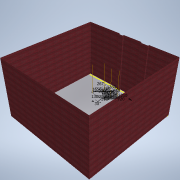
# Autodesk Inventor part: Entorno
Saved by Autodesk Inventor 2020 (Build 240168000, 168)
## iProperties
Created: 2019-10-05
Part Number: Entorno
Material: Genérico
Document SubType Name: Modeling
Designer: dasa1
Density: 1 g/cm^3
Appearance: Textura gruesa - Blanco
Author: dasa1
Autodesk Inventor part; units mm, degrees
ref_plane "YZ Plane" through (0, 0, 0) normal (1, 0, 0) x (0, 1, 0)
ref_plane "XZ Plane" through (0, 0, 0) normal (0, 1, 0) x (-1, 0, 0)
ref_plane "XY Plane" through (0, 0, 0) normal (0, 0, 1) x (1, 0, 0)
sketch "Boceto1" plane through (0, 0, 0) normal (0, 1, 0) x (-1, 0, 0)
  line L0 (0, 0) -> (0, -650) construction
  line L1 (0, -650) -> (4000, -650) construction
  line L2 (4000, -650) -> (-6000, -650)
  line L3 (-6000, -650) -> (-6000, 9350)
  line L4 (-6000, 9350) -> (4000, 9350)
  line L5 (4000, 9350) -> (4000, -650)
  dimension "d1" = 650
  dimension "d2" = 4000
  dimension "d3" = 10000
  dimension "d4" = 10000
  constraints: 12 end point, 2 parallel, 2 perpendicular, 1 horizontal, 1 vertical
  measures "d1" distance of L0.start L0.end
  measures "d2" distance of L0.end L1.end
  measures "d3" distance of L3.end L4.end
  measures "d4" distance of L2.end L3.end
extrude "Extrusión1" add sketch "Boceto1" along normal blind 1
sketch "Boceto3" plane through (0, 1, 0) normal (0, 1, 0) x (1, 0, 0)
  line L0 (-4000, 650) -> (-4000, -9350) construction
  line L1 (-4000, -9350) -> (6000, -9350) construction
  line L2 (6000, -9350) -> (6000, 650) construction
  line L3 (6000, 650) -> (-4000, 650) construction
  line L4 (6000, 650) -> (6000, 651)
  line L5 (-4000, 650) -> (-4000, -9350) projected
  line L6 (-4001, 650) -> (-4001, -9350)
  line L7 (-4001, -9350) -> (-4000, -9350)
  line L8 (-4000, -9350) -> (-4000, 650)
  line L9 (-4000, -9350) -> (6000, -9350)
  line L10 (6000, -9350) -> (6000, -9351)
  line L11 (6000, -9351) -> (-4000, -9351)
  line L12 (-4000, -9351) -> (-4000, -9350)
  line L13 (6000, -9350) -> (6001, -9350)
  line L14 (6001, -9350) -> (6001, 650)
  line L15 (6001, 650) -> (6000, 650) construction
  line L16 (6000, 650) -> (6000, -9350)
  line L17 (-50, 651) -> (200, 651)
  line L18 (200, 651) -> (-200, 651)
  line L19 (0, 651) -> (250, 651) construction
  line L20 (250, 651) -> (-249, 651) construction
  line L21 (-250, 651) -> (-249, 651) construction
  line L22 (-249, 651) -> (-249, 801)
  line L23 (-249, 801) -> (-250, 801)
  line L24 (-250, 800) -> (-250, 651)
  line L25 (250, 651) -> (249, 651) construction
  line L26 (249, 651) -> (249, 801)
  line L27 (249, 801) -> (250, 801)
  line L28 (250, 800) -> (250, 651)
  line L29 (249, 651) -> (-249, 651)
  line L30 (6000, 801) -> (6000, 800) construction
  line L31 (249, 800) -> (249, 801)
  line L32 (6001, 650) -> (6000, 650) construction
  line L33 (6000, 650) -> (6000, 800)
  line L34 (6000, 800) -> (6001, 800) construction
  line L35 (6001, 800) -> (6001, 650)
  line L36 (-250, 801) -> (-4000, 801)
  line L37 (-4000, 801) -> (-4000, 800) construction
  line L38 (-4000, 800) -> (-250, 800)
  line L39 (-250, 800) -> (-250, 801) construction
  line L40 (-4000, 801) -> (-4001, 801)
  line L41 (-4001, 801) -> (-4001, 650)
  line L42 (-4000, 651) -> (-4000, 800)
  line L43 (-250, 651) -> (-250, 650)
  line L44 (250, 651) -> (250, 650)
  line L45 (6000, 650) -> (-4000, 650) projected
  line L46 (6000, 801) -> (6001, 801)
  line L47 (6001, 801) -> (6001, 800)
  line L48 (6001, 800) -> (6000, 800) construction
  line L49 (6000, 800) -> (6000, 801) construction
  line L50 (2210, 650) -> (2210, 200) construction
  line L51 (2210, 200) -> (3040, 200) construction
  line L52 (3040, 200) -> (3040, 650) construction
  line L53 (3040, 650) -> (2210, 650) construction
  line L54 (2210, 650) -> (2211, 650)
  line L55 (2211, 651) -> (2211, 800)
  line L56 (2211, 800) -> (2210, 800) construction
  line L57 (2210, 800) -> (2210, 650)
  line L58 (3040, 650) -> (3039, 650)
  line L59 (3039, 651) -> (3039, 800)
  line L60 (3039, 800) -> (3040, 800) construction
  line L61 (3040, 800) -> (3040, 650)
  line L62 (2211, 650) -> (3039, 650)
  line L63 (3039, 650) -> (3039, 651) construction
  line L64 (3039, 651) -> (2211, 651)
  line L65 (2211, 651) -> (2211, 650) construction
  line L66 (2210, 800) -> (250, 800)
  line L67 (6000, 800) -> (3040, 800)
  line L68 (2211, 801) -> (2211, 800)
  line L69 (3039, 800) -> (3039, 801)
  line L70 (249, 801) -> (2211, 801)
  line L71 (3039, 801) -> (6000, 801)
  line L72 (-4000, 651) -> (-4000, 650)
  point P0 (0, 0)
  point P1 (-4000, -9350)
  point P2 (-4000, -9350)
  point P3 (-2000, -9350)
  point P4 (6000, 650)
  point P5 (6000, 650)
  dimension "d7" = 1
  dimension "d8" = 1
  dimension "d9" = 1
  dimension "d10" = 1
  dimension "d24" = 10000
  dimension "d32" = 0
  dimension "d34" = 0
  dimension "d36" = 10000
  dimension "d37" = 8000
  dimension "d38" = 10000
  dimension "d39" = 8000
  dimension "d40" = 10000
  dimension "d41" = 8000
  dimension "d42" = 0
  dimension "d81" = 250
  dimension "d82" = 500
  dimension "d83" = 1
  dimension "d84" = 150
  dimension "d85" = 1
  dimension "d86" = 150
  dimension "d87" = 1
  dimension "d88" = 1
  dimension "d89" = 90
  dimension "d90" = 90
  dimension "d94" = 0
  dimension "d95" = 0
  dimension "d96" = 151
  dimension "d97" = 5751
  dimension "d98" = 4250
  dimension "d99" = 0
  dimension "d100" = 1
  dimension "d101" = 0
  dimension "d102" = 0
  dimension "d103" = 150
  dimension "d104" = 5800
  dimension "d105" = 6050
  dimension "d106" = 0
  dimension "d107" = 1
  dimension "d108" = 0
  dimension "d111" = 1
  dimension "d112" = 1
  dimension "d113" = 1
  dimension "d114" = 90
  dimension "d115" = 151
  dimension "d116" = 150
  dimension "d117" = 2961
  constraints: 134 end point, 28 parallel, 16 perpendicular, 13 horizontal, 4 point on line, 1 collinear, 1 midpoint, 2 other
  measures "d7" distance of L4.end L4.start
  measures "d8" distance of L7.end L6.end
  measures "d9" distance of L9.end L10.end
  measures "d10" distance of L15.end L14.end
  measures "d24" distance between parallel lines of L3 L7
  measures "d32" distance from line of point (6000, 650) L3
  measures "d34" distance from line of point (6000, 650) L3
  measures "d36" distance from line of point (-4000, -9350) L3
  measures "d38" distance from line of point (-4000, -9350) L3
  measures "d40" distance from line of point (-2000, -9350) L3
  measures "d41" distance from line of point (-2000, -9350) L2
  measures "d42" distance between parallel lines of L2 L16
  measures "d81" distance of L19.start L19.end
  measures "d82" distance of L19.end L21.start
  measures "d83" distance of L23.end L22.end
  measures "d84" distance of L20.end L22.end
  measures "d85" distance of L26.end L27.end
  measures "d86" distance of L25.end L26.end
  measures "d87" distance of L30.start L30.end
  measures "d88" distance of L37.end L36.end
  measures "d89" angle to the sketch x axis of L44
  measures "d90" angle to the sketch x axis of L8
  measures "d94" vertical extent of L32
  measures "d95" distance between parallel lines of L2 L30
  measures "d96" distance between parallel lines of L3 L27
  measures "d97" distance between parallel lines of L2 L26
  measures "d98" distance between parallel lines of L0 L28
  measures "d99" distance between parallel lines of L0 L42
  measures "d100" distance from line of L4.end L3
  measures "d101" distance from line of point (6000, 650) L2
  measures "d102" distance from line of point (6000, 650) L2
  measures "d103" distance from line of L31.start L3
  measures "d104" distance from line of L17.end L2
  measures "d105" distance from line of L17.start L2
  measures "d106" distance from line of L43.end L3
  measures "d107" distance from line of L42.start L3
  measures "d108" distance from line of L6.start L3
  measures "d111" distance of L56.end L55.end
  measures "d112" distance of L59.end L60.end
  measures "d113" distance of L59.start L62.end
  measures "d114" angle of L53 L4
  measures "d115" distance between parallel lines of L53 L46
  measures "d116" distance between parallel lines of L53 L66
  measures "d117" distance from line of L58.end L2
extrude "Extrusión2" add sketch "Boceto3" along normal blind 6000 contours L4 L33 L67 L61 L45 L57 L66 L28 L44 L43 L24 L38 L42 L72 L5 L7 L6 L41 L40 L36 L23 L22 L29 L18 L17 L26 L27 L70 L68 L55 L64 L59 L69 L71 L46 L47 L35 L14 L13 L16 | L10 L11 L12 L9
sketch "Boceto4" plane through (0, 1, 0) normal (0, 1, 0) x (1, 0, 0)
  line L0 (0, 0) -> (370, 0) construction
  line L1 (0, 0) -> (2210, 0) construction
  line L2 (0, 0) -> (-385, 0) construction
  line L3 (0, 185) -> (0, 0) construction
  line L4 (0, 0) -> (-1260, 0) construction
  line L5 (0, 360) -> (0, 0) construction
  line L6 (0, 0) -> (250, 0) construction
  line L7 (250, 0) -> (250, -820) construction
  line L8 (250, -820) -> (0, -820) construction
  line L9 (0, -820) -> (0, 0) construction
  line L10 (0, 0) -> (-300, 0) construction
  line L11 (-300, 0) -> (-300, -1247) construction
  line L12 (-300, -1247) -> (0, -1247) construction
  line L13 (0, -1247) -> (0, 0) construction
  line L14 (0, 0) -> (30, 0) construction
  line L15 (30, 0) -> (30, -2220) construction
  line L16 (30, -2220) -> (0, -2220) construction
  line L17 (0, -2220) -> (0, 0) construction
  line L18 (0, 0) -> (1200, 0) construction
  line L19 (1200, 0) -> (1200, -720) construction
  line L20 (1200, -720) -> (0, -720) construction
  line L21 (0, -720) -> (0, 0) construction
  line L22 (0, 0) -> (-650, 0) construction
  line L23 (-650, 0) -> (-650, -650) construction
  line L24 (-650, -650) -> (0, -650) construction
  line L25 (0, -650) -> (0, 0) construction
  line L26 (6000, 650) -> (-4000, 650) projected
  line L27 (0, 0) -> (-1300, 0) construction
  line L28 (-1300, 0) -> (-1300, -1650) construction
  line L29 (-1300, -1650) -> (0, -1650) construction
  line L30 (0, -1650) -> (0, 0) construction
  line L31 (0, 0) -> (515, 0) construction
  line L32 (515, 0) -> (515, -1475) construction
  line L33 (515, -1475) -> (0, -1475) construction
  line L34 (0, -1475) -> (0, 0) construction
  line L35 (0, 0) -> (485, 0) construction
  line L36 (485, 0) -> (485, -1240) construction
  line L37 (485, -1240) -> (0, -1240) construction
  line L38 (0, -1240) -> (0, 0) construction
  line L39 (0, 0) -> (495, 0) construction
  line L40 (495, 0) -> (495, -972) construction
  line L41 (495, -972) -> (0, -972) construction
  line L42 (0, -972) -> (0, 0) construction
  line L43 (0, 0) -> (-385, 0) construction
  line L44 (-385, 0) -> (-385, -185) construction
  line L45 (-385, -185) -> (0, -185) construction
  line L46 (0, -185) -> (0, 0) construction
  line L47 (0, 0) -> (-1360, 0) construction
  line L48 (-1360, 0) -> (-1360, 267) construction
  line L49 (-1360, 267) -> (0, 267) construction
  line L50 (0, 267) -> (0, 0) construction
  line L51 (30, 0) -> (3030, 0) construction
  line L52 (0, 0) -> (-1414.2136, -1414.2136)
  line L53 (0, 0) -> (2000, 0) construction
  line L54 (0, 0) -> (30, -33.541)
  line L55 (30, -33.541) -> (-33.6396, 30.0986)
  line L56 (-33.6396, 30.0986) -> (-1447.8532, -1384.115)
  line L57 (-385, -185) -> (-1360, 0) construction
  point P0 (0, 650)
  dimension "d13" = 370
  dimension "d14" = 2210
  dimension "d19" = 250
  dimension "d20" = 820
  dimension "d21" = 300
  dimension "d22" = 1247
  dimension "d47" = 30
  dimension "d48" = 2220
  dimension "d49" = 1200
  dimension "d50" = 720
  dimension "d51" = 650
  dimension "d52" = 650
  dimension "d54" = 650
  dimension "d56" = 1300
  dimension "d57" = 1650
  dimension "d58" = 515
  dimension "d59" = 1475
  dimension "d60" = 485
  dimension "d61" = 1240
  dimension "d62" = 495
  dimension "d63" = 972
  dimension "d64" = 385
  dimension "d65" = 185
  dimension "d66" = 1360
  dimension "d67" = 267
  dimension "d70" = 2000
  dimension "d71" = 135
  dimension "d72" = 45
  dimension "d73" = 90
  dimension "d74" = 2000
  constraints: 82 end point, 30 horizontal, 22 parallel, 13 perpendicular, 13 vertical, 2 point on line, 1 coincident, 1 horizontal alignment, 6 other
  measures "d19" distance of L7.end L8.end
  measures "d20" distance of L6.end L7.end
  measures "d21" distance of L12.end L11.end
  measures "d22" distance of L11.end L10.end
  measures "d47" distance of L15.end L16.end
  measures "d48" distance of L14.end L15.end
  measures "d49" distance of L19.end L20.end
  measures "d50" distance of L18.end L19.end
  measures "d51" distance of L24.end L23.end
  measures "d52" distance of L23.end L22.end
  measures "d56" distance of L29.end L28.end
  measures "d57" distance of L28.end L27.end
  measures "d58" distance of L32.end L33.end
  measures "d59" distance of L31.end L32.end
  measures "d60" distance of L36.end L37.end
  measures "d61" distance of L35.end L36.end
  measures "d62" distance of L40.end L41.end
  measures "d63" distance of L39.end L40.end
  measures "d64" distance of L45.end L44.end
  measures "d65" distance of L44.end L43.end
  measures "d66" distance of L48.end L49.end
  measures "d67" distance of L47.end L48.end
  measures "d71" angle of L52 L53
  measures "d73" distance of L54.end L55.end
  measures "d74" distance of L55.end L56.end
sketch "Boceto5" plane through (0, 0, 0) normal (0, -1, 0) x (1, 0, 0)
  line L0 (-249, -801) -> (-4001, -801) projected
  line L1 (-249, -651) -> (-249, -801) projected
  line L2 (250, -650) -> (250, -800) projected
  line L3 (250, -800) -> (2210, -800) projected
  line L4 (2210, -800) -> (2210, -650) projected
  line L5 (6001, -801) -> (3039, -801) projected
  line L6 (3039, -801) -> (3039, -651) projected
  line L7 (6000, -800) -> (6000, -650) projected
  line L8 (-4000, -650) -> (-4000, -800) projected
  line L9 (6000, -650) -> (-4000, -650) projected
  line L10 (6001, -801) -> (3039, -801) projected
  line L11 (6000, -650) -> (3040, -650) projected
  line L12 (6001, -801) -> (3040, -801)
  line L13 (3040, -801) -> (3040, -650)
  line L14 (3040, -650) -> (6001, -650)
  line L15 (6001, -650) -> (6001, -801)
  line L16 (250, -800) -> (2210, -800) projected
  line L17 (249, -801) -> (249, -651) projected
  line L18 (2210, -800) -> (249, -800)
  line L19 (249, -800) -> (249, -651)
  line L20 (249, -651) -> (2210, -651)
  line L21 (2210, -651) -> (2210, -800)
  line L22 (-250, -650) -> (-4000, -650) projected
  line L23 (-249, -801) -> (-4000, -801)
  line L24 (-4000, -801) -> (-4000, -650)
  line L25 (-4000, -650) -> (-249, -650)
  line L26 (-249, -650) -> (-249, -801)
  point P0 (0, 0)
  point P1 (-249, -650)
  constraints: 24 end point, 6 parallel, 3 horizontal, 3 perpendicular
extrude "Extrusión3" add sketch "Boceto5" against normal blind 1 contours L9 L14 L15 L5 L13 | L0 L24 L8 L9 L26 L1 | L20 L4 L3 L2 | L2 L18 L17 L20
sketch "Boceto6" plane through (-249, 1, -650) normal (0, 0, 1) x (1, 0, 0)
  line L0 (499, 0) -> (0, 0) construction
  line L1 (499, 0) -> (499, 6000) construction
  line L2 (-1, 6000) -> (499, 6000) construction
  line L3 (-1, 0) -> (-1, 6000) construction
  line L4 (0, 0) -> (-1, 0) construction
  line L5 (249, -1) -> (249, 2299) construction
  line L6 (249, 2299) -> (249, 2449) construction
  line L7 (249, 2449) -> (249, 2661.5) construction
  line L8 (249, 2449) -> (289, 2449) construction
  line L9 (289, 2449) -> (289, 2474) construction
  line L10 (289, 2474) -> (249, 2474) construction
  line L11 (249, 2474) -> (249, 2449) construction
  line L12 (289, 2474) -> (209, 2474)
  line L13 (209, 2474) -> (209, 2449)
  line L14 (209, 2449) -> (289, 2449)
  line L15 (289, 2449) -> (289, 2474)
  line L16 (249, 2274) -> (289, 2274) construction
  line L17 (289, 2274) -> (289, 2299) construction
  line L18 (289, 2299) -> (249, 2299) construction
  line L19 (249, 2299) -> (249, 2274) construction
  line L20 (289, 2299) -> (209, 2299)
  line L21 (209, 2299) -> (209, 2274)
  line L22 (209, 2274) -> (289, 2274)
  line L23 (289, 2274) -> (289, 2299)
  line L24 (249, 2661.5) -> (274, 2661.5) construction
  line L25 (274, 2661.5) -> (274, 2674) construction
  line L26 (274, 2674) -> (249, 2674) construction
  line L27 (249, 2674) -> (249, 2661.5) construction
  line L28 (274, 2674) -> (224, 2674)
  line L29 (224, 2674) -> (224, 2649)
  line L30 (224, 2649) -> (274, 2649)
  line L31 (274, 2649) -> (274, 2674)
  line L32 (249, 2086.5) -> (274, 2086.5) construction
  line L33 (274, 2086.5) -> (274, 2099) construction
  line L34 (274, 2099) -> (249, 2099) construction
  line L35 (249, 2099) -> (249, 2086.5) construction
  line L36 (274, 2099) -> (224, 2099)
  line L37 (224, 2099) -> (224, 2074)
  line L38 (224, 2074) -> (274, 2074)
  line L39 (274, 2074) -> (274, 2099)
  dimension "d120" = 2300
  dimension "d121" = 150
  dimension "d122" = 212.5
  dimension "d125" = 40
  dimension "d126" = 25
  dimension "d127" = 80
  dimension "d128" = 25
  dimension "d129" = 40
  dimension "d130" = 25
  dimension "d131" = 80
  dimension "d132" = 25
  dimension "d135" = 25
  dimension "d136" = 12.5
  dimension "d137" = 50
  dimension "d138" = 25
  dimension "d142" = 25
  dimension "d143" = 12.5
  dimension "d144" = 50
  dimension "d145" = 25
  dimension "d164" = 2274
  dimension "d165" = 2099
  dimension "d166" = 210
  dimension "d167" = 225
  constraints: 70 end point, 16 parallel, 8 horizontal, 8 perpendicular, 3 vertical, 1 coincident
  measures "d120" distance of L5.start L5.end
  measures "d121" distance of L5.end L6.end
  measures "d122" distance of L6.end L7.end
  measures "d125" distance of L10.end L9.end
  measures "d126" distance of L9.end L8.end
  measures "d127" distance of L14.end L13.end
  measures "d128" distance of L13.end L12.end
  measures "d129" distance of L18.end L17.end
  measures "d130" distance of L17.end L16.end
  measures "d131" distance of L22.end L22.start
  measures "d132" distance of L22.start L20.end
  measures "d135" distance of L26.end L25.end
  measures "d136" distance of L25.end L24.end
  measures "d137" distance of L30.end L29.end
  measures "d138" distance of L29.end L28.end
  measures "d142" distance of L35.start L36.start
  measures "d143" distance of L36.start L32.end
  measures "d144" distance of L38.end L38.start
  measures "d145" distance of L38.start L37.start
  measures "d164" distance between parallel lines of L0 L16
  measures "d165" distance between parallel lines of L0 L34
  measures "d166" distance between parallel lines of L1 L17
  measures "d167" distance between parallel lines of L1 L33
extrude "Extrusión4" add sketch "Boceto6" along normal blind 80 contours L15 L14 L13 L12 | L23 L22 L21 L20
ref_plane "Plano de trabajo1" through (0, 2450, -650) normal (1, 0, 0) x (0, 1, 0)
sketch "Boceto7" plane through (0, 2450, -650) normal (1, 0, 0) x (0, 1, 0)
  line L0 (-2449, 0) -> (3551, 0) construction
  line L1 (25, 0) -> (25, 80) construction
  line L2 (0, 0) -> (0, 80) construction
  line L3 (-150, 0) -> (-150, 80) construction
  line L4 (-175, 0) -> (-175, 80) construction
  line L5 (-150, 0) -> (-150, 650) construction
  line L6 (-150, 0) -> (500, 0) construction
  line L7 (-150, 650) -> (-150, 0) construction
  line L8 (225, 0) -> (200, 0) construction
  line L9 (25, 0) -> (0, 0) construction
  line L10 (25, 0) -> (25, 80) construction
  line L11 (0, 80) -> (25, 80) construction
  line L12 (0, 0) -> (0, 80) construction
  line L13 (-150, 0) -> (-175, 0) construction
  line L14 (-150, 0) -> (-150, 80) construction
  line L15 (-175, 80) -> (-150, 80) construction
  line L16 (-175, 0) -> (-175, 80) construction
  line L17 (-350, 0) -> (-375, 0) construction
  line L18 (-2449, 10000) -> (-2449, -150) construction
  line L19 (-2449, -150) -> (3551, -150) construction
  line L20 (3551, 10000) -> (3551, -150) construction
  line L21 (-2449, 10000) -> (3551, 10000) construction
  line L22 (-150, 80) -> (-175, 80)
  line L23 (-175, 80) -> (-175, 700)
  line L24 (-175, 700) -> (-150, 700)
  line L25 (-150, 700) -> (-150, 80)
  line L26 (25, 0) -> (25, 650) construction
  line L27 (25, 650) -> (25, 0) construction
  line L28 (25, 80) -> (0, 80)
  line L29 (0, 80) -> (0, 700)
  line L30 (0, 700) -> (25, 700)
  line L31 (25, 700) -> (25, 80)
  line L32 (25, 650) -> (25, 600) construction
  line L33 (-150, 650) -> (-150, 600) construction
  line L34 (225, 0) -> (25, 600)
  line L35 (200, 0) -> (25, 525)
  line L36 (-350, 0) -> (-175, 525)
  line L37 (-375, 0) -> (-350, 0)
  line L38 (-375, 0) -> (-175, 600)
  line L39 (200, 0) -> (225, 0)
  line L40 (-350, 0) -> (-375, 0)
  line L41 (225, 0) -> (-375, 0)
  line L42 (-375, 0) -> (-350, 0)
  line L43 (-175, 600) -> (-175, 525)
  line L44 (-350, 0) -> (-375, 0)
  line L45 (225, 0) -> (200, 0)
  line L46 (-375, 0) -> (-350, 0)
  line L47 (-175, 600) -> (-175, 525)
  point P0 (-2450, 650)
  point P1 (25, 525)
  point P2 (25, 600)
  dimension "d139" = 650
  dimension "d140" = 90
  dimension "d150" = 25
  dimension "d151" = 620
  dimension "d152" = 650
  dimension "d153" = 25
  dimension "d154" = 620
  dimension "d155" = 50
  dimension "d156" = 18.435
  dimension "d157" = 18.435
  dimension "d158" = 3526
  dimension "d159" = 3526
  dimension "d160" = 700
  dimension "d161" = 600
  constraints: 62 end point, 6 parallel, 5 collinear, 5 point on line, 3 horizontal, 3 perpendicular, 2 vertical
  measures "d139" distance of L3.start L5.end
  measures "d140" angle of L6 L5
  measures "d150" distance of L23.end L24.end
  measures "d151" distance of L22.end L23.end
  measures "d152" distance of L26.start L26.end
  measures "d153" distance of L29.end L31.start
  measures "d154" distance of L29.start L29.end
  measures "d155" distance of L26.end L32.end
  measures "d156" angle of L20 L34
  measures "d157" angle of L20 L36
  measures "d158" distance between parallel lines of L20 L31
  measures "d159" distance between parallel lines of L20 L26
  measures "d160" distance between parallel lines of L8 L30
  measures "d161" distance from line of L33.end L8
sketch "Boceto8" plane through (-249, 1, -650) normal (0, 0, 1) x (1, 0, 0)
  line L0 (249, 2674) -> (249, 3174) construction
  line L1 (289, 2474) -> (289, 2449) construction
  line L2 (289, 2449) -> (209, 2449) construction
  line L3 (209, 2449) -> (209, 2474) construction
  line L4 (209, 2474) -> (289, 2474) construction
  line L5 (289, 2299) -> (289, 2274) construction
  line L6 (289, 2274) -> (209, 2274) construction
  line L7 (209, 2274) -> (209, 2299) construction
  line L8 (209, 2299) -> (289, 2299) construction
  line L9 (499, 0) -> (0, 0) construction
  line L10 (499, 0) -> (499, 6000) construction
  line L11 (-1, 6000) -> (499, 6000) construction
  line L12 (-1, 0) -> (-1, 6000) construction
  line L13 (0, 0) -> (-1, 0) construction
  line L14 (0, -1) -> (0, 6000) construction
  line L15 (249, 3174) -> (0, 3174) construction
  line L16 (0, 3174) -> (0, 3214) construction
  line L17 (0, 3214) -> (249, 3214) construction
  line L18 (249, 3214) -> (249, 3174) construction
  line L19 (498, 0) -> (498, 6000) projected
  line L20 (0, 3174) -> (498, 3174)
  line L21 (498, 3174) -> (498, 3214)
  line L22 (498, 3214) -> (0, 3214)
  line L23 (0, 3214) -> (0, 3174)
  point P0 (249, -1)
  dimension "d146" = 500
  dimension "d147" = 40
  dimension "d173" = 3214
  dimension "d174" = 3214
  dimension "d175" = 250
  dimension "d176" = 3174
  dimension "d177" = 1
  constraints: 18 end point, 4 parallel, 2 horizontal, 2 perpendicular, 2 point on line, 1 vertical
  measures "d146" distance of L0.start L0.end
  measures "d147" distance of L15.end L16.end
  measures "d173" distance between parallel lines of L9 L22
  measures "d174" distance between parallel lines of L9 L17
  measures "d175" distance between parallel lines of L10 L0
  measures "d176" distance from line of point (498, 3174) L9
  measures "d177" distance from line of point (498, 3174) L10
extrude "Extrusión5" add sketch "Boceto8" along normal blind 20
extrude "Extrusión6" add sketch "Boceto7" along normal mid plane 80
sketch "Boceto9" plane through (-249, 3215, -650) normal (0, 1, 0) x (1, 0, 0)
  line L0 (0, -20) -> (498, -20) projected
  line L1 (249, -20) -> (269, -20)
  line L2 (269, -20) -> (229, -20)
  line L3 (229, -20) -> (269, -20)
  line L4 (269, -20) -> (269, -820)
  line L5 (269, -820) -> (229, -820)
  line L6 (229, -820) -> (229, -20)
  line L7 (498, -20) -> (458, -20) construction
  line L8 (0, -20) -> (40, -20) construction
  line L9 (498, -20) -> (0, -20) projected
  line L10 (229, -20) -> (229, -420) construction
  line L11 (229, -420) -> (269, -420) construction
  line L12 (40, -20) -> (80, -20)
  line L13 (458, -20) -> (418, -20)
  line L14 (40, -20) -> (229, -420)
  line L15 (80, -20) -> (229, -335.3439)
  line L16 (418, -20) -> (269, -335.3439)
  line L17 (458, -20) -> (269, -420)
  point P0 (249, -650)
  point P1 (418, -20)
  point P2 (269, -20)
  point P3 (229, -20)
  point P4 (229, -335.3439)
  point P5 (80, -20)
  point P6 (40, -20)
  dimension "d168" = 20
  dimension "d169" = 40
  dimension "d170" = 0
  dimension "d171" = 40
  dimension "d172" = 800
  dimension "d178" = 40
  dimension "d179" = 40
  dimension "d180" = 400
  dimension "d181" = 40
  dimension "d182" = 40
  constraints: 32 end point, 4 parallel, 4 point on line, 3 midpoint, 1 collinear, 1 horizontal, 1 perpendicular, 4 other
  measures "d168" distance of L1.start L1.end
  measures "d169" distance of L1.end L2.end
  measures "d170" distance between parallel lines of L2 L1
  measures "d171" distance of L4.end L5.end
  measures "d172" distance of L3.end L4.end
  measures "d178" distance of L0.end L7.end
  measures "d179" distance of L0.start L8.end
  measures "d180" distance of L2.end L10.end
  measures "d181" distance of L8.end L12.end
  measures "d182" distance of L7.end L13.end
extrude "Extrusión7" add sketch "Boceto9" against normal blind 40 contours L0 L15 L6 L14 | L6 L0 L4 L5 | L4 L16 L0 L17
sketch "Boceto10" plane through (20, 3215, 170) normal (1, 0, 0) x (0, 0, -1)
  line L0 (0, 0) -> (400, 0) construction
  line L1 (0, 0) -> (0, -40) construction
  line L2 (400, -40) -> (0, -40) construction
  line L3 (400, 0) -> (400, -40) construction
  line L4 (820, -540) -> (220, -740) construction
  line L5 (820, -740) -> (820, -765) construction
  line L6 (820, -740) -> (295, -740) construction
  line L7 (295, -740) -> (820, -565) construction
  line L8 (820, -540) -> (820, -565) construction
  line L9 (820, -540) -> (220, -740) construction
  line L10 (220, -740) -> (120, -740) construction
  line L11 (120, -740) -> (120, -765) construction
  line L12 (820, -765) -> (120, -765) construction
  line L13 (0, -40) -> (400, -40) projected
  line L14 (220, -740) -> (820, -540) projected
  line L15 (502.759, -647.7642) -> (466.759, -659.7642)
  line L16 (400, -40) -> (0, -40) projected
  line L17 (0, 0) -> (400, 0) projected
  line L18 (260.171, -40) -> (300.171, -40)
  line L19 (340.171, -40) -> (322.6308, -40)
  line L20 (260.171, -40) -> (466.759, -659.7642)
  line L21 (300.171, -40) -> (502.759, -647.7642)
  line L22 (322.6308, -40) -> (522.9729, -641.0262)
  line L23 (340.171, -40) -> (538.759, -635.7642)
  line L24 (466.1539, -657.9487) -> (538.1539, -633.9487)
  point P0 (170, -3215)
  point P1 (522.3677, -639.2108)
  dimension "d198" = 1.9137
  dimension "d199" = 16.6401
  dimension "d200" = 37.9473
  dimension "d201" = 75.8947
  dimension "d202" = 297.0919
  dimension "d203" = 1.9137
  dimension "d204" = 1.9137
  constraints: 16 end point, 8 point on line, 4 perpendicular, 1 parallel
  measures "d198" distance between parallel lines of L9 L15
  measures "d199" distance between parallel lines of L23 L22
  measures "d200" distance between parallel lines of L23 L21
  measures "d201" distance between parallel lines of L23 L20
  measures "d202" distance from line of L4.start L23
  measures "d203" distance from line of L23.end L14
  measures "d204" distance from line of L22.end L9
extrude "Extrusión8" add sketch "Boceto10" against normal blind 40 contours L13 L21 L14 L20 | L14 L21 L15 L20 | L13 L23 L14 L22
fillet "Empalme1" radius 8.32 4 edges at (-20, 2875.3946, -252.4993) (-20, 2878.0256, -269.1624) (20, 2878.0256, -269.1624) (20, 2875.3946, -252.4993)
sketch "Boceto11" plane through (-249, 3215, -650) normal (0, 1, 0) x (1, 0, 0)
  line L0 (0, 0) -> (498, 0) projected
  line L1 (498, 0) -> (498, -20) projected
  line L2 (0, 0) -> (498, 0)
  line L3 (498, 0) -> (498, -20)
  line L4 (498, -20) -> (0, -20)
  line L5 (0, -20) -> (0, 0)
  point P0 (249, -650)
  constraints: 8 end point, 2 parallel, 1 horizontal, 1 perpendicular
extrude "Extrusión9" add sketch "Boceto11" along normal blind 20
sketch "Boceto12" plane through (-249, 3175, -650) normal (0, -1, 0) x (1, 0, 0)
  line L0 (0, 0) -> (498, 0) projected
  line L1 (269, 20) -> (418, 20) projected
  line L2 (229, 488.5991) -> (229, 420) projected
  line L3 (229, 420) -> (40, 20) projected
  line L4 (0, 20) -> (40, 20) projected
  line L5 (0, 0) -> (0, 20) projected
  line L6 (498, 0) -> (0, 0) projected
  line L7 (498, 0) -> (498, 20) projected
  line L8 (458, 20) -> (498, 20) projected
  line L9 (458, 20) -> (269, 420) projected
  line L10 (269, 559.829) -> (269, 820) projected
  line L11 (269, 20) -> (418, 20) projected
  line L12 (269, 20) -> (269, 335.3439) projected
  line L13 (269, 335.3439) -> (418, 20) projected
  line L14 (80, 20) -> (229, 20) projected
  line L15 (80, 20) -> (229, 335.3439) projected
  line L16 (229, 335.3439) -> (229, 20) projected
  line L17 (458, 20) -> (498, 20) projected
  line L18 (498, 0) -> (0, 0) projected
  line L19 (498, 20) -> (0, 20)
  line L20 (0, 20) -> (0, 0)
  line L21 (0, 0) -> (498, 0)
  line L22 (498, 0) -> (498, 20)
  line L23 (269, 820) -> (229, 820) projected
  line L24 (237.32, 497.3692) -> (260.68, 497.3692) projected
  line L25 (269, 488.5991) -> (269, 519.829) projected
  line L26 (269, 519.829) -> (229, 519.829) projected
  line L27 (229, 519.829) -> (229, 488.5991) projected
  line L28 (260.68, 479.829) -> (237.32, 479.829) projected
  line L29 (269, 420) -> (269, 488.5991) projected
  line L30 (229, 559.829) -> (269, 559.829) projected
  line L31 (229, 820) -> (229, 559.829) projected
  ellipse E0 centre (260.68, 488.5991) end of major axis (260.68, 479.8291) minor radius 8.32 (269, 488.5991) -> (260.68, 497.3692) ccw projected
  ellipse E1 centre (237.32, 488.5991) end of major axis (237.32, 479.8291) minor radius 8.32 (237.32, 497.3692) -> (229, 488.5991) ccw projected
  ellipse E2 centre (237.32, 488.5991) end of major axis (237.32, 497.3691) minor radius 8.32 (229, 488.5991) -> (237.32, 479.829) ccw projected
  ellipse E3 centre (260.68, 488.5991) end of major axis (260.68, 497.3691) minor radius 8.32 (260.68, 479.829) -> (269, 488.5991) ccw projected
  point P0 (249, 650)
  point P1 (80, 20)
  point P2 (40, 20)
  point P3 (458, 20)
  point P4 (418, 20)
  point P5 (269, 20)
  point P6 (229, 20)
  constraints: 8 end point, 2 parallel, 1 horizontal, 1 perpendicular, 4 other
extrude "Extrusión10" add sketch "Boceto12" along normal blind 20 contours L5 L4 L19 L14 L1 L8 L7 L0
sketch "Boceto13" plane through (-40, 2300, -650) normal (0, 1, 0) x (1, 0, 0)
  circle A0 centre (40, -650) radius 25
  dimension "d193" = 50
  constraints: 1 centre point, 1 coincident
  measures "d193" diameter of A0
extrude "Extrusión11" cut sketch "Boceto13" along normal blind 200 and the other way blind 50
sketch "Boceto14" plane through (-20, 3175, 170) normal (0, -1, 0) x (1, 0, 0)
  point P0 (20, -170)
sketch "Boceto15" plane through (0, 2450, -650) normal (1, 0, 0) x (0, 1, 0)
  line L0 (128.4203, 289.7392) -> (725, 488.5991) construction
  line L1 (128.4203, 289.7392) -> (128.4203, 289.7392) construction
  line L2 (725, 488.5991) -> (128.4203, 289.7392) construction
  line L3 (725, 420) -> (725, 488.5991) construction
  line L4 (765, 420) -> (725, 420) construction
  line L5 (765, 820) -> (765, 420) construction
  line L6 (765, 820) -> (725, 820) construction
  line L7 (725, 559.829) -> (725, 820) construction
  line L8 (725, 559.829) -> (107.0513, 353.8461) construction
  line L9 (119.0513, 317.8461) -> (107.0513, 353.8461) construction
  line L10 (119.0513, 317.8461) -> (725, 519.829) construction
  line L11 (725, 488.5991) -> (725, 519.829) construction
  line L12 (725, 820) -> (725, 559.829) construction
  line L13 (725, 559.829) -> (725, 820) construction
  line L14 (725, 650) -> (714, 650)
  line L15 (714, 650) -> (714, 667.5)
  line L16 (714, 667.5) -> (725, 667.5)
  line L17 (725, 667.5) -> (725, 650)
  line L18 (714, 650) -> (706, 650)
  line L19 (706, 650) -> (706, 658)
  line L20 (706, 658) -> (714, 658)
  line L21 (714, 658) -> (714, 650)
  line L22 (706, 650) -> (695, 650)
  line L23 (695, 650) -> (695, 667.5)
  line L24 (695, 667.5) -> (706, 667.5)
  line L25 (706, 667.5) -> (706, 650)
  point P0 (-2450, 650)
  point P1 (714, 658)
  point P2 (706, 658)
  dimension "d211" = 11
  dimension "d212" = 17.5
  dimension "d213" = 8
  dimension "d214" = 8
  dimension "d215" = 11
  dimension "d216" = 17.5
  constraints: 24 end point, 6 parallel, 3 horizontal, 3 perpendicular, 1 point on line
  measures "d211" distance of L15.end L16.end
  measures "d212" distance of L14.end L15.end
  measures "d213" distance of L19.end L20.end
  measures "d214" distance of L18.end L19.end
  measures "d215" distance of L23.end L24.end
  measures "d216" distance of L22.end L23.end
revolve "Revolución1" add sketch "Boceto15" angle 360 about axis through (0, 3175, 0) along (0, -1, 0)
